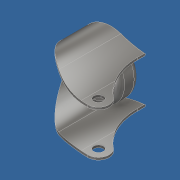
# Autodesk Inventor part: Axel Mount
Saved by Autodesk Inventor 2018 (Build 220112000, 112)
## iProperties
Created: 2018-03-27
Part Number: Axel Mount
Material: Steel, Alloy
Document SubType Name: Modeling
Designer: Cole
Density: 7.73 g/cm^3
Appearance: Semi-Polished
Author: Cole
Autodesk Inventor part; units mm, degrees
ref_plane "YZ Plane" through (0, 0, 0) normal (1, 0, 0) x (0, 1, 0)
ref_plane "XZ Plane" through (0, 0, 0) normal (0, 1, 0) x (-1, 0, 0)
ref_plane "XY Plane" through (0, 0, 0) normal (0, 0, 1) x (1, 0, 0)
sketch "Sketch1" plane through (0, 0, 0) normal (0, 0, 1) x (1, 0, 0)
  circle A0 centre (0, 0) radius 7.493
  circle A1 centre (0, 0) radius 24.13
  dimension "d0" = 14.986
  dimension "d1" = 48.26
  constraints: 2 centre point, 2 coincident
  measures "d0" diameter of A0
  measures "d1" diameter of A1
extrude "Extrusion1" add sketch "Sketch1" along normal blind 17.78
fillet "Fillet1" radius 4.7625 2 edges at (-24.13, 0, 17.78) (-24.13, 0, 0)
sketch "Sketch2" plane through (0, 0, 0) normal (0, 0, -1) x (-1, 0, 0)
  circle A0 centre (0, 0) radius 24.13 projected
  arc A1 (-8.7661, -24.6497) -> (26.162, 0) centre (0, 0) ccw
  line L0 (-36.8072, -17.78) -> (-52.07, -17.78)
  arc A2 (-8.0852, -22.7351) -> (-36.8072, -17.78) centre (-36.8072, -103.4997) ccw
  line L1 (-52.07, -19.812) -> (-36.8072, -19.812)
  arc A3 (-8.7661, -24.6497) -> (-36.8072, -19.812) centre (-36.8072, -103.4997) ccw
  arc A4 (-8.0852, -22.7351) -> (-8.0852, 22.7351) centre (0, 0) ccw
  line L2 (-52.07, -17.78) -> (-52.07, -19.812)
  circle A5 centre (0, 0) radius 7.493 projected
  arc A6 (26.162, 0) -> (-8.7661, 24.6497) centre (0, 0) ccw
  line L3 (-36.8072, 17.78) -> (-52.07, 17.78)
  arc A7 (-36.8072, 17.78) -> (-8.0852, 22.7351) centre (-36.8072, 103.4997) ccw
  line L4 (-52.07, 19.812) -> (-36.8072, 19.812)
  arc A8 (-36.8072, 19.812) -> (-8.7661, 24.6497) centre (-36.8072, 103.4997) ccw
  line L5 (-52.07, 17.78) -> (-52.07, 19.812)
  circle A9 centre (0, 0) radius 7.493
  line L6 (7.493, 0) -> (-7.493, 0)
  dimension "d5" = 2.032
  dimension "d8" = 17.78
  dimension "d9" = 2.032
  dimension "d10" = 52.07
  constraints: 16 point on circle, 14 end point, 8 centre point, 2 coincident, 2 horizontal, 1 tangent, 1 vertical, 5 other
  measures "d8" distance from line of A1.centre L0
  measures "d9" distance between parallel lines of L0 L1
  measures "d10" distance from line of A5.centre L2
extrude "Extrusion2" add sketch "Sketch2" against normal blind 63.5 contours A0 A7 L3 L5 L4 A8 A6 A1 A3 L1 L2 L0 A2
ref_plane "Work Plane2" through (36.8072, 32.512, 0) normal (0, 1, 0) x (1, 0, 0)
sketch "Sketch4" plane through (36.8072, 32.512, 0) normal (0, 1, 0) x (1, 0, 0)
  line L0 (0, 0) -> (15.2628, 0) projected
  line L1 (0, 0) -> (0, -63.5) projected
  line L2 (15.2628, -63.5) -> (0, -63.5) projected
  line L3 (15.2628, 0) -> (15.2628, -63.5) projected
  line L4 (-28.0411, 0) -> (0, 0) projected
  line L5 (-28.0411, 0) -> (-28.0411, -63.5) projected
  line L6 (0, -63.5) -> (-28.0411, -63.5) projected
  line L7 (0, 0) -> (0, -63.5) projected
  line L8 (-28.0411, 0) -> (-28.0411, 0) projected
  line L9 (-28.0411, 0) -> (-28.0411, -63.5) projected
  line L10 (-28.0411, -63.5) -> (-28.0411, -63.5) projected
  line L11 (-28.0411, 0) -> (-28.0411, -63.5) projected
  line L12 (-28.722, -63.5) -> (0, -63.5) projected
  circle A0 centre (6.0934, -54.3306) radius 4.0894
  arc A1 (6.0934, -63.5) -> (11.781, -47.1382) centre (6.0934, -54.3306) ccw
  arc A2 (-7.5972, -7.1097) -> (11.781, -47.1382) centre (43.4345, -7.1097) ccw
  line L13 (-17.4397, -17.78) -> (-56.1747, -17.78) projected
  arc A3 (-60.9372, -13.0175) -> (-56.1747, -17.78) centre (-56.1747, -13.0175) ccw projected
  arc A4 (-17.4397, -17.78) -> (-12.6772, -13.0175) centre (-17.4397, -13.0175) ccw projected
  line L14 (-12.6772, -4.7625) -> (-12.6772, -13.0175) projected
  line L15 (-62.9692, 0) -> (-62.9692, -63.5) projected
  line L16 (0, -63.5) -> (15.2628, -63.5) projected
  arc A5 (-56.6375, -23.3247) -> (6.0934, -63.5) centre (6.0934, 5.5626) ccw
  arc A6 (-56.6375, -23.3247) -> (-62.9692, -13.7244) centre (-91.2445, -39.261) ccw
  line L17 (-7.5972, 0) -> (-7.5972, -7.1097)
  line L18 (-7.5972, -62.1294) -> (-7.5972, -63.5)
  line L19 (-7.5972, 0) -> (-7.5972, 40.7656)
  line L20 (-7.5972, 40.7656) -> (62.5891, 40.1908)
  line L21 (62.5891, 40.1908) -> (61.5259, -89.632)
  line L22 (61.5259, -89.632) -> (-86.4704, -80.382)
  line L23 (-86.4704, -80.382) -> (-75.0747, -4.7625)
  line L24 (-75.0747, -4.7625) -> (-62.9692, -13.7244)
  point P0 (-36.8072, 0)
  point P1 (-59.3182, -16.5952)
  dimension "d15" = 22.86
  dimension "d16" = 8.1788
  dimension "d17" = 9.1694
  dimension "d18" = 9.1694
  dimension "d19" = 5.08
  dimension "d22" = 38.1
  constraints: 16 end point, 11 point on circle, 6 tangent, 5 centre point, 4 point on line, 3 perpendicular, 1 vertical
  measures "d15" distance from line of L3 L17.start
  measures "d16" diameter of A0
  measures "d17" distance from line of L2 A0.centre
  measures "d18" distance from line of L3 A0.centre
  measures "d19" radial gap between concentric circles of A0 A1
  measures "d22" radius of A6
extrude "Extrusion3" cut sketch "Sketch4" against normal blind 63.5 contours L4 L19 L20 L21 L22 L23 L24 A6 A5 L5 L6 L2 L3 L0 | L0 L3 A1 A2 L1 | L1 A2 L17 L4 | L3 L2 A1 | A5 L2 L1 | L1 L6 L18 A5 | L18 L6 L5 A5 | A0
full round fillet "Fillet2" first side at (6.7418, -25.2784, 34.9927) centre faces at (12.8404, -21.9741, 0) second side at (6.2498, -23.3066, 1.5875)
equation "\"d18\" = d17"
body "Solid1"
